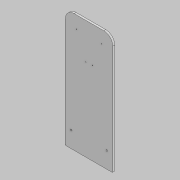
# Autodesk Inventor part: mountPlate
Saved by Autodesk Inventor 2020 (Build 240168000, 168)
## iProperties
Created: 2020-07-21
Part Number: mountPlate
Material: Generic
Document SubType Name: Modeling
Designer: lu0248
Density: 1 g/cm^3
Appearance: Default
Author: lu0248
Autodesk Inventor part; units mm, degrees
ref_plane "YZ Plane" through (0, 0, 0) normal (1, 0, 0) x (0, 1, 0)
ref_plane "XZ Plane" through (0, 0, 0) normal (0, 1, 0) x (-1, 0, 0)
ref_plane "XY Plane" through (0, 0, 0) normal (0, 0, 1) x (1, 0, 0)
sketch "Sketch1" plane through (0, 0, 0) normal (0, 0, 1) x (1, 0, 0)
  line L0 (-120, 0) -> (120, 0)
  line L1 (120, 0) -> (120, 600)
  line L2 (120, 600) -> (-120, 600)
  line L3 (-120, 600) -> (-120, 0)
  point P0 (0, 0)
  dimension "d0" = 600
  dimension "d1" = 240
  dimension "d2" = 120
  constraints: 8 end point, 2 parallel, 1 horizontal, 1 midpoint, 1 perpendicular
  measures "d0" distance of L2.end L0.start
  measures "d1" distance of L1.end L2.end
  measures "d2" distance from line of point (0, 0) L3
extrude "Extrusion1" add sketch "Sketch1" along normal blind 10
fillet "Fillet1" radius 45 2 edges at (120, 600, 5) (-120, 600, 5)
sketch "Sketch2" plane through (0, 0, 10) normal (0, 0, 1) x (1, 0, 0)
  line L0 (-120, 555) -> (-120, 0) projected
  line L1 (120, 0) -> (120, 555) projected
  line L2 (-120, 0) -> (120, 0) projected
  point P0 (0, 0)
  point P1 (-90, 82)
  point P2 (90, 82)
  dimension "d8" = 82
  dimension "d9" = 82
  dimension "d17" = 90
  dimension "d18" = 90
  measures "d8" distance from line of L2 point (90, 82)
  measures "d9" distance from line of L2 point (-90, 82)
  measures "d17" horizontal distance of point (0, 0) point (90, 82)
  measures "d18" horizontal distance of point (0, 0) point (-90, 82)
hole "Hole1" at (-90, 82, 10) at (90, 82, 10) direction (0, 0, -1) diameter 8 depth 60
sketch "Sketch3" plane through (0, 0, 10) normal (0, 0, 1) x (1, 0, 0)
  line L0 (75, 600) -> (-75, 600) projected
  point P0 (0, 0)
  point P1 (-63.5, 537.035)
  point P2 (63.5, 537.035)
  point P3 (-17, 416.8674)
  point P4 (17, 418.5659)
  dimension "d19" = 17
  dimension "d20" = 17
  dimension "d21" = 63.5
  dimension "d22" = 63.5
  dimension "d23" = 62.965
  dimension "d24" = 62.965
  dimension "d25" = 120.1676
  dimension "d26" = 118.4691
  measures "d19" horizontal distance of point (0, 0) point (-17, 416.867)
  measures "d20" horizontal distance of point (0, 0) point (17, 418.566)
  measures "d21" horizontal distance of point (0, 0) point (-63.5, 537.035)
  measures "d22" horizontal distance of point (0, 0) point (63.5, 537.035)
  measures "d23" distance from line of L0 point (-63.5, 537.035)
  measures "d24" distance from line of L0 point (63.5, 537.035)
  measures "d25" vertical distance of point (-63.5, 537.035) point (-17, 416.867)
  measures "d26" vertical distance of point (63.5, 537.035) point (17, 418.566)
hole "Hole2" at (17, 418.5659, 10) at (-17, 416.8674, 10) at (63.5, 537.035, 10) at (-63.5, 537.035, 10) direction (0, 0, -1) diameter 4 end through all
fillet "Fillet2" radius 2 2 edges at (-120, 0, 5) (120, 0, 5)
equation "\"d0\" = partHeight"
equation "\"d1\" = partWidth"
equation "\"d2\" = 0.5 * partWidth"
equation "\"d3\" = thickness"
equation "\"d8\" = holeHeight"
equation "\"d9\" = holeHeight"
equation "\"d17\" = 0.5 * ribThickness + 0.5 * ribSpacing"
equation "\"d18\" = 0.5 * ribThickness + 0.5 * ribSpacing"
equation "\"d19\" = 0.5 * lowerHoleSpacing"
equation "\"d20\" = 0.5 * lowerHoleSpacing"
equation "\"d21\" = 0.5 * upperHoleSpacing"
equation "\"d22\" = 0.5 * upperHoleSpacing"
equation "\"d27\" = mountHoleDiameter"
equation "\"partWidth\" = 240"
equation "\"partHeight\" = 600"
equation "\"thickness\" = 10"
equation "\"holeHeight\" = 82"
equation "\"upperHoleSpacing\" = 127"
equation "\"lowerHoleSpacing\" = 34"
equation "\"mountHoleDiameter\" = 4"
equation "\"ribThickness\" = 20"
equation "\"ribSpacing\" = 160"
body "Solid1"
